shat from morot to coupler v1 (Autodesk Fusion 360 design; units mm, degrees)
Autodesk Fusion 360 part; units mm, degrees
note: some values were not read from the file. Set by a fixed rule: which sketch regions a step uses.
sketch "Sketch1" plane through (0, 0, 0) normal (0, 0, 1) x (1, 0, 0)
  circle A0 centre (0, 0) radius 14
  dimension "d1" = 28
  constraint coincident A0.centre origin
  measures "d1" diameter of A0
extrude "Extrude1" add sketch "Sketch1" along normal blind 120
sketch "Sketch2" plane through (0, 0, 120) normal (0, 0, 1) x (1, 0, 0)
  circle A0 centre (0, 0) radius 14
  line L0 (0, 0) -> (0, 0.5314)
  line L1 (0, 0.5314) -> (0, 14)
  line L2 (0, 14) -> (-4, 14)
  line L3 (-4, 14) -> (-4, 10)
  line L4 (4, 10) -> (-4, 10)
  line L5 (0, 14) -> (4, 14)
  line L6 (4, 14) -> (4, 10)
  dimension "d4" = 8
  dimension "d5" = 4
  dimension "d6" = 4
  dimension "d7" = 4
  constraint coincident A0.centre L0.start
  constraint vertical L0
  constraint coincident A0 L1.end
  constraint parallel L0 L1
  constraint perpendicular L1 L2
  constraint perpendicular L2 L3
  constraint perpendicular L3 L4
  constraint perpendicular L1 L5
  constraint perpendicular L4 L6
  measures "d4" distance of L3.end L4.start
  measures "d5" distance of L4.start L5.end
  measures "d6" distance of L1 L6
  measures "d7" distance of L1 L3
extrude "Extrude2" cut sketch "Sketch2" along normal blind -120 and the other way blind 5 contours A0 L1 L4 L6 | A0 L1 L3 L4
sketch "Sketch3" plane through (0, 0, 120) normal (0, 0, 1) x (1, 0, 0)
  circle A0 centre (0, 0) radius 11
  circle A1 centre (0, 0) radius 14
  dimension "d10" = 22
  constraint concentric A0 A1
  measures "d10" diameter of A0
extrude "Extrude4" add sketch "Sketch3" along normal blind 40 contours A0
extrude "Extrude3" add sketch "Sketch3" along normal blind 40 contours A0
sketch "Sketch4" plane through (0, 0, 160) normal (0, 0, 1) x (1, 0, 0)
  circle A0 centre (0, 0) radius 11
  line L0 (0, 0) -> (0, 11)
  line L1 (0, 11) -> (-2.5, 11)
  line L2 (0, 11) -> (2.5, 11)
  line L3 (-2.5, 11) -> (-2.5, 8)
  line L4 (-2.5, 8) -> (2.5, 8)
  line L5 (2.5, 11) -> (2.5, 8)
  dimension "d17" = 2.5
  dimension "d18" = 2.5
  dimension "d19" = 90
  dimension "d20" = 3
  constraint coincident A0.centre L0.start
  constraint coincident A0 L0.end
  constraint vertical L0
  constraint perpendicular L0 L1
  constraint horizontal L2
  constraint perpendicular L1 L3
  constraint perpendicular L0 L4
  measures "d17" distance of L0.end L1.end
  measures "d18" distance of L0.end L2.end
  measures "d19" angle of L4 L5
  measures "d20" distance of L2.end L4.end
extrude "Extrude5" cut sketch "Sketch4" against normal blind 35 contours A0 L0 L4 L5 | A0 L0 L3 L4
fillet "Fillet1" radius 2.5 2 edges at (2.5, 9.3561, 125) (-2.5, 9.3561, 125)
fillet "Fillet2" radius 4 2 edges at (4, 11.7082, 115) (-4, 11.7082, 115)
